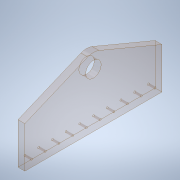
# Autodesk Inventor part: Jeep Plate 2.0
Saved by Autodesk Inventor 2020 (Build 240168000, 168)
## iProperties
Created: 2020-02-14
Part Number: Jeep Plate 2.0
Material: Polycarbonate, Smoke
Document SubType Name: Modeling
Designer: aidan
Density: 1.2 g/cm^3
Appearance: Polycarbonate - Smoked
Author: aidan
Autodesk Inventor part; units mm, degrees
ref_plane "YZ Plane" through (0, 0, 0) normal (1, 0, 0) x (0, 1, 0)
ref_plane "XZ Plane" through (0, 0, 0) normal (0, 1, 0) x (-1, 0, 0)
ref_plane "XY Plane" through (0, 0, 0) normal (0, 0, 1) x (1, 0, 0)
sketch "Sketch1" plane through (0, 0, 0) normal (1, 0, 0) x (0, 1, 0)
  line L0 (127, 254) -> (0, 254)
  line L1 (0, 254) -> (0, 0)
  line L2 (0, 0) -> (127, 0)
  line L3 (127, 0) -> (127, 254)
  circle A0 centre (100.0125, 127) radius 14.2875
  circle A1 centre (100.0125, 127) radius 26.9875
  line L4 (76.2, 254) -> (124.914, 137.4039)
  line L5 (124.914, 116.5961) -> (76.2, 0)
  dimension "d0" = 254
  dimension "d1" = 127
  dimension "d2" = 28.575
  dimension "d3" = 12.7
  dimension "d4" = 127
  dimension "d5" = 76.2
  dimension "d6" = 76.2
  constraints: 12 end point, 2 centre point, 2 coincident, 2 parallel, 2 point on circle, 2 point on line, 2 tangent, 1 equal length, 1 horizontal, 1 perpendicular
  measures "d0" distance of L2.end L0.start
  measures "d1" distance of L0.start L0.end
  measures "d2" diameter of A0
  measures "d3" radial gap between concentric circles of A0 A1
  measures "d4" distance from line of L0 A0.centre
  measures "d5" distance from line of L1 L5.end
  measures "d6" distance from line of L1 L4.start
extrude "Extrusion1" add sketch "Sketch1" along normal blind 12.7 contours L4 A1 L5 L2 L1 L0 | A1
sketch "Sketch2" plane through (12.7, 0, 0) normal (1, 0, 0) x (0, 0, -1)
  circle A0 centre (-241.3, 12.7) radius 1.7272
  line L0 (-254, 76.2) -> (-254, 0) projected
  line L1 (-254, 0) -> (0, 0) projected
  dimension "d9" = 12.7
  dimension "d10" = 12.7
  dimension "d11" = 3.4544
  constraints: 1 centre point
  measures "d9" distance from line of L0 A0.centre
  measures "d10" distance from line of L1 A0.centre
  measures "d11" diameter of A0
extrude "Extrusion2" cut sketch "Sketch2" against normal through all
pattern_linear "Rectangular Pattern1" count 10 spacing 25.4 along (0, 0, -1) of "Extrusion2"
body "Solid1"
